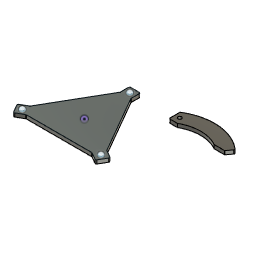
Hook Wheel Parts v1 (Autodesk Fusion 360 design; units mm, degrees)
Autodesk Fusion 360 part; units mm, degrees
sketch "Sketch1" plane through (0, 0, 0) normal (0, 0, 1) x (1, 0, 0)
  line L0 (0, 0) -> (140, 0) construction
  line L1 (-106.2269, -44.0096) -> (-15, 114)
  line L2 (15, 114) -> (106.2269, -44.0096)
  line L3 (91.2269, -69.9904) -> (-91.2269, -69.9904)
  line L4 (-15, 140) -> (15, 140)
  line L5 (15, 140) -> (15, 114)
  line L6 (-15, 114) -> (-15, 140)
  line L7 (15, 140) -> (14.2708, 139.2708) construction
  line L8 (-128.7436, -57.0096) -> (-106.2269, -44.0096)
  line L9 (-113.7436, -82.9904) -> (-128.7436, -57.0096)
  line L10 (-91.2269, -69.9904) -> (-113.7436, -82.9904)
  line L11 (113.7436, -82.9904) -> (91.2269, -69.9904)
  line L12 (128.7436, -57.0096) -> (113.7436, -82.9904)
  line L13 (106.2269, -44.0096) -> (128.7436, -57.0096)
  dimension "d5" = 30
  dimension "d6" = 26
  dimension "d7" = 26
  dimension "d8" = 26
  dimension "d9" = 30
  dimension "d10" = 26
  dimension "d11" = 30
  dimension "d12" = 26
  dimension "d13" = 26
  constraint horizontal L0
  constraint coincident L0.start origin
  constraint horizontal L3
  constraint horizontal L4
  constraint perpendicular L4 L5
  constraint parallel L5 L6
  measures "d5" distance of L4.start L4.end
  measures "d6" distance of L4.end L2.start
  measures "d7" distance of L4.start L1.end
  measures "d8" distance of L12.start L2.end
  measures "d9" distance of L11.start L12.start
  measures "d10" distance of L11.start L3.start
  measures "d11" distance of L8.start L9.start
  measures "d12" distance of L8.start L1.start
  measures "d13" distance of L9.start L3.end
extrude "Extrude1" add sketch "Sketch1" along normal blind 10 makes body 1
fillet "Fillet1" radius 3 12 edges at (-113.7436, -82.9904, 5) (-91.2269, -69.9904, 5) (91.2269, -69.9904, 5) (113.7436, -82.9904, 5) (-128.7436, -57.0096, 5) (-106.2269, -44.0096, 5) (-15, 114, 5) (-15, 140, 5) (15, 140, 5) (15, 114, 5) (106.2269, -44.0096, 5) (128.7436, -57.0096, 5) on bodies 1
sketch "Sketch2" plane through (0, 0, 0) normal (0, 0, 1) x (1, 0, 0)
  line L0 (240.6616, 203.5291) -> (270, 203.5291)
  line L1 (270, 203.5291) -> (282.3476, 220.2232)
  line L2 (139.3384, 203.5291) -> (115.9466, 203.5291)
  line L3 (115.9466, 203.5291) -> (115.9466, 233.8111)
  arc A0 (240.6616, 203.5291) -> (139.3384, 203.5291) centre (190, 115) ccw
  arc A1 (282.3476, 220.2232) -> (115.9466, 233.8111) centre (190, 115) ccw
  dimension "d18" = 280
  constraint horizontal L0
  constraint parallel L0 L2
  constraint perpendicular L2 L3
  constraint concentric A0 A1
  measures "d18" diameter of A1
extrude "Extrude2" add sketch "Sketch2" along normal blind 10 separate body makes body 2
fillet "Fillet2" radius 3 2 edges at (115.9466, 203.5291, 5) (282.3476, 220.2232, 5) on bodies 2
sketch "Sketch3" plane through (0, 0, 10) normal (0, 0, 1) x (-1, 0, 0)
  arc A0 (-127.2436, 59.6077) -> (-126.1455, 55.5096) centre (-124.6455, 58.1077) ccw
  line L0 (-126.1455, 55.5096) -> (-106.9231, 44.4115)
  arc A1 (-105.825, 43.3134) -> (-106.9231, 44.4115) centre (-108.4231, 41.8134) ccw
  line L1 (-105.825, 43.3134) -> (-15.4019, -113.3038)
  arc A2 (-15, -114.8038) -> (-15.4019, -113.3038) centre (-18, -114.8038) ccw
  line L2 (-15, -114.8038) -> (-15, -137)
  arc A3 (-15, -137) -> (-12, -140) centre (-12, -137) ccw
  line L3 (-12, -140) -> (12, -140)
  arc A4 (12, -140) -> (15, -137) centre (12, -137) ccw
  line L4 (15, -137) -> (15, -114.8038)
  arc A5 (15.4019, -113.3038) -> (15, -114.8038) centre (18, -114.8038) ccw
  line L5 (15.4019, -113.3038) -> (105.825, 43.3134)
  arc A6 (106.9231, 44.4115) -> (105.825, 43.3134) centre (108.4231, 41.8134) ccw
  line L6 (106.9231, 44.4115) -> (126.1455, 55.5096)
  arc A7 (126.1455, 55.5096) -> (127.2436, 59.6077) centre (124.6455, 58.1077) ccw
  line L7 (127.2436, 59.6077) -> (115.2436, 80.3923)
  arc A8 (115.2436, 80.3923) -> (111.1455, 81.4904) centre (112.6455, 78.8923) ccw
  line L8 (111.1455, 81.4904) -> (91.923, 70.3923)
  arc A9 (90.423, 69.9904) -> (91.923, 70.3923) centre (90.423, 72.9904) ccw
  line L9 (90.423, 69.9904) -> (-90.423, 69.9904)
  arc A10 (-91.923, 70.3923) -> (-90.423, 69.9904) centre (-90.423, 72.9904) ccw
  line L10 (-91.923, 70.3923) -> (-111.1455, 81.4904)
  arc A11 (-111.1455, 81.4904) -> (-115.2436, 80.3923) centre (-112.6455, 78.8923) ccw
  line L11 (-115.2436, 80.3923) -> (-127.2436, 59.6077)
  circle A12 centre (0, -125.9019) radius 5
  circle A13 centre (109.0343, 62.951) radius 5
  circle A14 centre (-109.0343, 62.951) radius 5
  dimension "d24" = 10
  dimension "d28" = 360
  measures "d24" diameter of A12
extrude "Extrude3" cut sketch "Sketch3" against normal blind 10 contours A12 bodies 1
extrude "Extrude4" cut sketch "Sketch3" against normal blind 10 contours A13 bodies 1
extrude "Extrude5" cut sketch "Sketch3" against normal blind 10 contours A14 bodies 1
move_body "Move1" bodies 2 to x (1, 0, 0) y (0, 1, 0) z (0, 0, 1) at (0, -85, 0)
sketch "Sketch4" plane through (0, 0, 10) normal (0, 0, 1) x (-1, 0, 0)
  arc A0 (-280.6901, -132.9823) -> (-280.2113, -137.0604) centre (-278.2782, -134.7663) ccw
  arc A1 (-280.2113, -137.0604) -> (-115.9466, -148.8111) centre (-190, -30) ccw
  line L0 (-115.9466, -148.8111) -> (-115.9466, -121.5291)
  arc A2 (-115.9466, -121.5291) -> (-118.9466, -118.5291) centre (-118.9466, -121.5291) ccw
  line L1 (-118.9466, -118.5291) -> (-139.3384, -118.5291)
  arc A3 (-240.6616, -118.5291) -> (-139.3384, -118.5291) centre (-190, -30) ccw
  line L2 (-240.6616, -118.5291) -> (-270, -118.5291)
  line L3 (-270, -118.5291) -> (-280.6901, -132.9823)
  circle A4 centre (-129.1425, -135.1701) radius 5
  dimension "d33" = 10
  measures "d33" diameter of A4
extrude "Extrude6" cut sketch "Sketch4" against normal blind 10 contours A4 bodies 2
fillet "Fillet3" radius 1 2 edges at (240.6616, 118.5291, 5) (270, 118.5291, 5) on bodies 2
